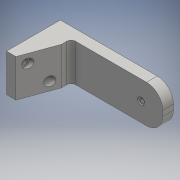
# Autodesk Inventor part: Large Bracket (RHS)
Saved by Autodesk Inventor 2016 (Build 200138000, 138)
## iProperties
Created: 2018-10-20
Part Number: Large Bracket (RHS)
Material: Generic
Document SubType Name: Modeling
Designer: DML
Density: 1 g/cm^3
Appearance: Default
Author: DML
Autodesk Inventor part; units mm, degrees
ref_plane "YZ Plane" through (0, 0, 0) normal (1, 0, 0) x (0, 1, 0)
ref_plane "XZ Plane" through (0, 0, 0) normal (0, 1, 0) x (-1, 0, 0)
sketch "Sketch1" plane through (0, 0, 0) normal (0, 1, 0) x (-1, 0, 0)
  line L0 (0, 0) -> (105, 0)
  line L1 (105, 0) -> (105, -35)
  line L2 (105, -35) -> (0, -35)
  line L3 (0, -35) -> (0, 0)
  dimension "d0" = 35
  dimension "d1" = 105
  constraints: 8 end point, 2 parallel, 1 horizontal, 1 perpendicular
  measures "d0" distance of L2.end L0.start
  measures "d1" distance of L0.start L0.end
extrude "Extrusion1" add sketch "Sketch1" along normal blind 10
sketch "Sketch2" plane through (0, 10, 0) normal (0, 1, 0) x (1, 0, 0)
  circle A0 centre (-20, 17.5) radius 11.25
  line L0 (0, 35) -> (-105, 35) projected
  line L1 (-105, 35) -> (-105, 0) projected
  point P0 (0, 0)
  dimension "d4" = 22.5
  dimension "d5" = 17.5
  dimension "d6" = 85
  constraints: 1 centre point
  measures "d4" diameter of A0
  measures "d5" distance from line of L0 A0.centre
  measures "d6" distance from line of A0.centre L1
extrude "Extrusion2" cut sketch "Sketch2" against normal blind 5
sketch "Sketch3" plane through (0, 0, 0) normal (0, -1, 0) x (1, 0, 0)
  circle A0 centre (-20, -17.5) radius 11.25 construction
  point P0 (0, 0)
  constraints: 2 coincident
hole "Hole1" at (-20, 0, -17.5) direction (0, 1, 0) diameter 4 depth 8 tip angle 118 counterbore diameter 6.5 counterbore depth 1
sketch "Sketch4" plane through (0, 0, 0) normal (0, -1, 0) x (1, 0, 0)
  line L0 (-105, -35) -> (0, -35) projected
  line L1 (-105, -35) -> (-85, -35)
  line L2 (-85, -35) -> (-85, 0)
  line L3 (-85, 0) -> (-105, 0)
  line L4 (-105, 0) -> (-105, -35)
  point P0 (0, 0)
  dimension "d16" = 20
  constraints: 8 end point, 2 parallel, 1 horizontal, 1 perpendicular
  measures "d16" distance of L2.end L3.end
extrude "Extrusion3" add sketch "Sketch4" along normal blind 40
sketch "Sketch5" plane through (-105, 10, 0) normal (0, 0, 1) x (1, 0, 0)
  line L0 (20, -50) -> (0, -50) projected
  line L1 (8.7445, -50) -> (20, -19.0668)
  line L2 (20, -10) -> (20, -50) projected
  line L3 (20, -50) -> (8.7445, -50)
  line L4 (20, -50) -> (20, -19.0668)
  point P0 (105, -10)
  constraints: 6 end point, 2 collinear, 2 point on line
extrude "Extrusion4" cut sketch "Sketch5" against normal blind 42
ref_plane "Work Plane1" through (-85, 10, -35) normal (-1, 0, 0) x (0, 0, 1)
sketch "Sketch6" plane through (-85, 10, -35) normal (-1, 0, 0) x (0, 0, 1)
  circle A0 centre (27, -42) radius 4.25
  line L0 (35, -50) -> (35, -19.0668) projected
  line L1 (0, -50) -> (35, -50) projected
  circle A1 centre (8, -27.0668) radius 4.25
  line L2 (35, -19.0668) -> (0, -19.0668) projected
  line L3 (0, -19.0668) -> (0, -50) projected
  point P0 (35, -10)
  dimension "d22" = 8.5
  dimension "d23" = 8
  dimension "d24" = 8
  dimension "d25" = 8.5
  dimension "d26" = 8
  dimension "d27" = 8
  constraints: 2 centre point
  measures "d22" diameter of A0
  measures "d23" distance from line of L0 A0.centre
  measures "d24" distance from line of L1 A0.centre
  measures "d25" diameter of A1
  measures "d26" distance from line of A1.centre L2
  measures "d27" distance from line of L3 A1.centre
extrude "Extrusion5" cut sketch "Sketch6" along normal blind 11 contours A0 | A1
sketch "Sketch7" plane through (-96, -32, -8) normal (1, 0, 0) x (0, 0, -1)
  point P0 (-8, 32)
  point P1 (0, 0)
hole "Hole2" at (-96, -32, -8) direction (-1, 0, 0) diameter 4.5 depth 10 tip angle 118
sketch "Sketch8" plane through (-96, -17.0668, -27) normal (1, 0, 0) x (0, 0, -1)
  point P0 (-27, 17.0668)
  point P1 (0, 0)
hole "Hole3" at (-96, -17.0668, -27) direction (-1, 0, 0) diameter 4.5 depth 10 tip angle 118
fillet "Fillet1" radius 4 1 edges at (-85, 0, -17.5)
fillet "Fillet2" radius 15 1 edges at (0, 5, 0)
fillet "Fillet3" radius 15 1 edges at (0, 5, -35)
body "Solid1"
